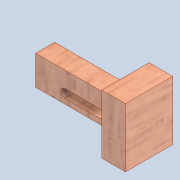
# Autodesk Inventor part: 0005-10-025 Activator senzor Y
Saved by Autodesk Inventor 2020 (Build 240168000, 168)
## iProperties
Created: 2020-12-18
Part Number: 0005-10-025 Activator senzor Y
Material: Generic
Document SubType Name: Modeling
Designer: Iulian Bors
Density: 1 g/cm^3
Appearance: White Oak - Natural Medium Gloss
Author: Iulian Bors
Subject: 025
Autodesk Inventor part; units mm, degrees
ref_plane "YZ Plane" through (0, 0, 0) normal (1, 0, 0) x (0, 1, 0)
ref_plane "XZ Plane" through (0, 0, 0) normal (0, 1, 0) x (-1, 0, 0)
ref_plane "XY Plane" through (0, 0, 0) normal (0, 0, 1) x (1, 0, 0)
sketch "Sketch1" plane through (0, 0, 0) normal (0, 0, 1) x (1, 0, 0)
  line L0 (-25, 12.5) -> (25, 12.5)
  line L1 (25, 12.5) -> (25, -12.5)
  line L2 (25, -12.5) -> (-25, -12.5)
  line L3 (-25, -12.5) -> (-25, 12.5)
  point P0 (0, 0)
  point P1 (0, 12.5)
  point P2 (-25, 0)
  dimension "d0" = 50
  dimension "d1" = 25
  constraints: 8 end point, 2 midpoint, 2 parallel, 1 horizontal, 1 horizontal alignment, 1 perpendicular, 1 vertical alignment
  measures "d0" distance of L0.start L0.end
  measures "d1" distance of L2.end L0.start
extrude "Extrusion1" add sketch "Sketch1" along normal blind 20
sketch "Sketch5" plane through (0, 0, 20) normal (0, 0, 1) x (1, 0, 0)
  line L0 (2.5, 8.5) -> (-12.5, 8.5) construction
  line L1 (2.5, 10.25) -> (-12.5, 10.25)
  line L2 (-12.5, 6.75) -> (2.5, 6.75)
  arc A0 (2.5, 6.75) -> (2.5, 10.25) centre (2.5, 8.5) ccw
  arc A1 (-12.5, 10.25) -> (-12.5, 6.75) centre (-12.5, 8.5) ccw
  line L3 (2.5, -8.5) -> (-12.5, -8.5) construction
  line L4 (2.5, -6.75) -> (-12.5, -6.75)
  line L5 (-12.5, -10.25) -> (2.5, -10.25)
  arc A2 (2.5, -10.25) -> (2.5, -6.75) centre (2.5, -8.5) ccw
  arc A3 (-12.5, -6.75) -> (-12.5, -10.25) centre (-12.5, -8.5) ccw
  line L6 (25, 12.5) -> (-25, 12.5) projected
  line L7 (-25, -12.5) -> (25, -12.5) projected
  line L8 (-25, 12.5) -> (-25, -12.5) projected
  point P0 (0, 0)
  point P1 (-5, 8.5)
  point P2 (-5, -8.5)
  dimension "d29" = 3.5
  dimension "d30" = 4
  dimension "d31" = 4
  dimension "d32" = 20
  dimension "d33" = 15
  constraints: 16 end point, 8 point on circle, 8 tangent, 5 parallel, 4 centre point, 2 midpoint, 1 equal radius, 1 horizontal, 1 vertical alignment
  measures "d29" distance between parallel lines of L2 L1
  measures "d30" distance between parallel lines of L0 L6
  measures "d31" distance between parallel lines of L7 L3
  measures "d32" distance from line of L8 point (-5, 8.5)
  measures "d33" distance of L0.start L0.end
extrude "Extrusion5" cut sketch "Sketch5" against normal through all contours A2 L5 A3 L4
sketch "Sketch6" plane through (0, 0, 20) normal (0, 0, 1) x (1, 0, 0)
  line L0 (15, 0) -> (-25, 0)
  line L1 (-25, 0) -> (-25, 12.5)
  line L2 (-25, 12.5) -> (15, 12.5)
  line L3 (15, 12.5) -> (15, 0)
  line L4 (25, -12.5) -> (25, 12.5) projected
  line L5 (-25, 12.5) -> (-25, -12.5) projected
  line L6 (25, 12.5) -> (-25, 12.5) projected
  point P0 (0, 0)
  dimension "d36" = 10
  constraints: 8 end point, 2 collinear, 2 parallel, 1 horizontal, 1 perpendicular, 1 point on line
  measures "d36" distance between parallel lines of L3 L4
extrude "Extrusion6" cut sketch "Sketch6" against normal through all
sketch "Sketch7" plane through (0, 0, 20) normal (0, 0, 1) x (1, 0, 0)
  line L0 (15, -12.5) -> (-25, -12.5)
  line L1 (-25, -12.5) -> (-25, 0)
  line L2 (-25, 0) -> (15, 0)
  line L3 (15, 0) -> (15, -12.5)
  line L4 (15, 12.5) -> (15, 0) projected
  line L5 (-25, -12.5) -> (25, -12.5) projected
  line L6 (-25, 0) -> (-25, -12.5) projected
  line L7 (15, 0) -> (-25, 0) projected
  point P0 (0, 0)
  point P1 (15, 2)
  point P2 (13, 0)
  constraints: 8 end point, 4 collinear, 2 parallel, 1 horizontal, 1 perpendicular
extrude "Extrusion7" cut sketch "Sketch7" against normal blind 12
fillet "Fillet2" radius 2 1 edges at (15, 0, 4)
body "Solid1"
